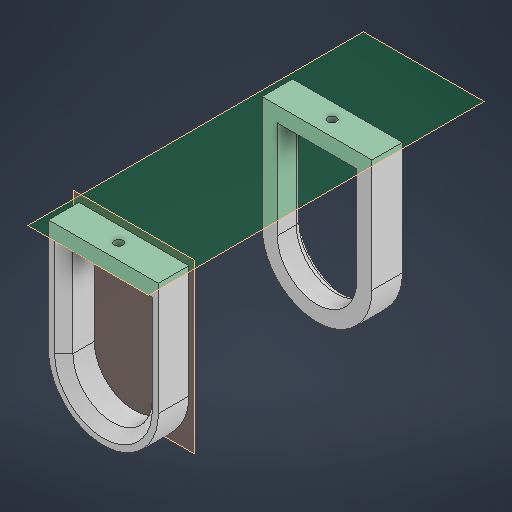
# Autodesk Inventor part: Payload Mount
Saved by Autodesk Inventor 2026.1 (Build 301233000, 233)
## iProperties
Created: 2026-03-28
Part Number: Payload Mount
Material: Generic
Document SubType Name: Modeling
Designer: elisa
Density: 1 g/cm^3
Appearance: Default
Author: elisa
Autodesk Inventor part; units mm, degrees
ref_plane "YZ Plane" through (0, 0, 0) normal (1, 0, 0) x (0, 1, 0)
ref_plane "XZ Plane" through (0, 0, 0) normal (0, 1, 0) x (-1, 0, 0)
ref_plane "XY Plane" through (0, 0, 0) normal (0, 0, 1) x (1, 0, 0)
sketch "Sketch1" plane through (0, 0, 0) normal (0, 0, 1) x (1, 0, 0)
  line L0 (170.0568, 0) -> (-170.0568, 0) construction
  line L1 (-170.0568, -123.761) -> (170.0568, -123.761) construction
  arc A0 (-26, -74) -> (26, -74) centre (0, -74) ccw
  line L2 (26, -10) -> (-26, -10)
  line L3 (-26, -74) -> (-26, -10)
  line L4 (-26, 0) -> (-26, 0)
  line L5 (26, -74) -> (26, -10)
  line L6 (26, 0) -> (26, 0)
  line L7 (-36, 0) -> (36, 0)
  line L8 (36, 0) -> (36, -74)
  arc A1 (-36, -74) -> (36, -74) centre (0, -74) ccw
  line L9 (-36, -74) -> (-36, 0)
  point P0 (0, 0)
  point P1 (0, -100)
  point P2 (0, 0)
  dimension "d0" = 123.761
  dimension "d3" = 26
  dimension "d7" = 90
  dimension "d22" = 10
  constraints: 20 end point, 5 point on circle, 4 perpendicular, 4 tangent, 2 centre point, 2 horizontal, 2 point on line, 1 coincident, 1 midpoint, 3 other
  measures "d0" distance between parallel lines of L1 L0
  measures "d3" radius of A0
  measures "d7" distance from line of point (0, -100) L2
  measures "d22" distance between parallel lines of L3 L9
extrude "Rear Support" add sketch "Sketch1" along normal blind 20
ref_plane "Support Spacing" through (0, 0, 140) normal (0, 0, 1) x (1, 0, 0)
sketch "Sketch5" plane through (0, 0, 140) normal (0, 0, 1) x (1, 0, 0)
  line L0 (36, -74) -> (36, 0) projected
  line L1 (36, 0) -> (-36, 0) projected
  line L2 (-36, 0) -> (-36, -74) projected
  arc A0 (-36, -74) -> (36, -74) centre (0, -74) ccw projected
  line L3 (-26, -74) -> (-26, -10) projected
  line L4 (-26, -10) -> (26, -10) projected
  line L5 (26, -10) -> (26, -74) projected
  arc A1 (-26, -74) -> (26, -74) centre (0, -74) ccw projected
  point P0 (0, 0)
extrude "Front Support" add sketch "Sketch5" along normal blind 20
sketch "Sketch6" plane through (-26, -10, 140) normal (0, -1, 0) x (1, 0, 0)
  line L0 (62, 0) -> (62, 20) construction
  line L1 (62, 10) -> (-10, 10) construction
  line L2 (-10, 0) -> (-10, 20) construction
  line L3 (0, 0) -> (52, 0) construction
  line L4 (26, 0) -> (26, 20) construction
  line L5 (62, 20) -> (-10, 20) construction
  line L6 (62, -140) -> (62, -120) construction
  line L7 (62, -130) -> (-10, -130) construction
  line L8 (-10, -140) -> (-10, -120) construction
  line L9 (26, -140) -> (26, -120) construction
  line L10 (0, -120) -> (52, -120) construction
  circle A0 centre (26, 10) radius 4.5
  circle A1 centre (26, -130) radius 4.5
  dimension "d25" = 9
  constraints: 9 midpoint, 8 end point, 2 centre point
  measures "d25" diameter of A0
extrude "Screw Head" cut sketch "Sketch6" against normal blind 5.5
sketch "Sketch7" plane through (-36, 0, 140) normal (0, 1, 0) x (1, 0, 0)
  circle A0 centre (36, -10) radius 4.5 projected
  circle A1 centre (36, -10) radius 2.75
  circle A2 centre (36, 130) radius 4.5 projected
  circle A3 centre (36, 130) radius 2.75
  point P0 (36, 140)
  dimension "d28" = 5.5
  constraints: 2 centre point, 2 coincident
  measures "d28" diameter of A1
extrude "Screw Thread" cut sketch "Sketch7" against normal blind 10 contours A1 | A3
chamfer "Dual Chamfer" distance 6 angle 45 6 edges at (0, -100, 0) (-26, -42, 0) (26, -42, 0) (0, -100, 160) (-26, -42, 160) (26, -42, 160)
chamfer "Top Exit Chamfer" distance 5 distance2 9 1 edges at (0, -10, 140) measured on face at (0, -10, 140.5)
fillet "Rear Fillet" radius 4 6 edges at (-32, -42, 0) (32, -42, 0) (0, -106, 0) (26, -42, 6) (-26, -42, 6) (0, -100, 6)
ref_plane "Fuselage Bottom" through (36, 0, 160) normal (0, -1, 0) x (-1, 0, 0)
body "Solid1"
